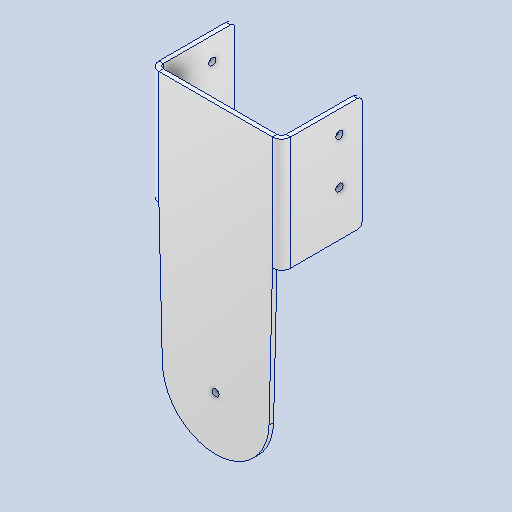
# Autodesk Inventor part: servoplate2_forR3
Saved by Autodesk Inventor 2024.3 (Build 283343010, 343A)
## iProperties
Created: 2025-05-28
Part Number: servoplate2_forR3
Material: アルミニウム 6061
Document SubType Name: Sheet Metal
Designer: kshau
Density: 2.7 g/cm^3
Sheet Metal Rule: Default
Appearance: アルミニウム - フラット
Mass: 54.6317 g
Surface Area: 213.118 cm^2
Volume: 20.234 cm^3
Flat Pattern Width: 13.35 cm
Flat Pattern Length: 12.2048 cm
Flat Pattern Area: 162.934 cm^2
Sheet Metal Width: 133.500 mm
Sheet Metal Length: 122.048 mm
Sheet Metal Area: 16293.380 mm^2
Author: kshau
Autodesk Inventor part; units mm, degrees
ref_plane "YZ Plane" through (0, 0, 0) normal (1, 0, 0) x (0, 1, 0)
ref_plane "XZ Plane" through (0, 0, 0) normal (0, 1, 0) x (-1, 0, 0)
ref_plane "XY Plane" through (0, 0, 0) normal (0, 0, 1) x (1, 0, 0)
sketch "スケッチ1" plane through (0, 0, 0) normal (0, 0, 1) x (1, 0, 0)
  circle A0 centre (0, 0) radius 23.5
  line L0 (0, 0) -> (0, 60)
  line L1 (0, 60) -> (25, 60)
  line L2 (25, 60) -> (25, 110)
  line L3 (25, 110) -> (0, 110)
  line L4 (0, 110) -> (0, 60)
  line L5 (25, 60) -> (23.4927, -0.5845)
  line L6 (0, 60) -> (-25, 60)
  line L7 (-25, 60) -> (-25, 110)
  line L8 (-25, 110) -> (0, 110)
  line L9 (-25, 60) -> (-23.4927, -0.5845)
  point P0 (-23.4927, -0.5845)
  dimension "d0" = 47
  dimension "d1" = 60
  dimension "d2" = 50
  dimension "d3" = 25
  measures "d1" distance of L0.start L0.end
  measures "d2" distance of L1.end L2.end
  measures "d3" distance of L0.end L1.end
extrude "プレート1" add sketch "スケッチ1" along normal blind 2
sketch "スケッチ2" plane through (27, 60, -2) normal (1, 0, 0) x (0, 1, 0)
  line L0 (50, 0) -> (0, 0)
  line L1 (0, 0) -> (0, -31.5)
  line L2 (0, -31.5) -> (50, -31.5)
  line L3 (50, -31.5) -> (50, 0)
  constraints: 6 end point, 1 horizontal, 1 perpendicular, 1 vertical
edge flange "フランジ1" height 35.5 angle 90 thickness 2 bend radius 2 thickness toward (1, 0, 0) relief straight relief width 2 relief depth 1 edges at (25, 85, 0) wall of the first edge with corners at (27, 110, -2) (27, 60, -2) (27, 60, -33.5) (27, 110, -33.5)
bend "曲げ1"
corner "コーナー1"
sketch "スケッチ3" plane through (-27, 110, -2) normal (-1, 0, 0) x (0, -1, 0)
  line L0 (50, 0) -> (0, 0)
  line L1 (0, 0) -> (0, -31.5)
  line L2 (0, -31.5) -> (50, -31.5)
  line L3 (50, -31.5) -> (50, 0)
  constraints: 6 end point, 1 horizontal, 1 perpendicular, 1 vertical
edge flange "フランジ2" height 35.5 angle 90 thickness 2 bend radius 2 thickness toward (-1, 0, 0) relief straight relief width 2 relief depth 1 edges at (-25, 85, 0) wall of the first edge with corners at (-27, 60, -2) (-27, 110, -2) (-27, 110, -33.5) (-27, 60, -33.5)
bend "曲げ2"
corner "コーナー2"
sketch "スケッチ4" plane through (0, 0, 2) normal (0, 0, 1) x (1, 0, 0)
  circle A0 centre (0, 0) radius 10.1
  dimension "d25" = 20.2
  constraints: 1 centre point, 1 coincident
  measures "d25" diameter of A0
extrude "押し出し1" [suppressed]
sketch "スケッチ5" plane through (0, 0, 2) normal (0, 0, 1) x (1, 0, 0)
  circle A0 centre (0, 0) radius 15.18
  point P0 (0, 15.18)
  point P1 (-13.1463, 7.59)
  point P2 (-13.1463, -7.59)
  point P3 (0, -15.18)
  point P4 (13.1463, -7.59)
  point P5 (13.1463, 7.59)
  dimension "d28" = 30.36
  dimension "d31" = 360
  constraints: 1 coincident, 1 vertical alignment, 9 other
hole "穴1" [suppressed]
sketch "スケッチ6" plane through (29, 60, -33.5) normal (1, 0, 0) x (0, 0, -1)
  line L0 (0, 0) -> (0, 50) projected
  line L1 (0, 10) -> (-31.5, 10)
  line L2 (-31.5, 50) -> (-31.5, 0) projected
  line L3 (0, 0) -> (-31.5, 0) projected
  line L4 (0, 50) -> (-31.5, 50) projected
  line L5 (-10, 50) -> (-10, 10)
  point P0 (-33.5, -60)
  point P1 (-10, 20)
  point P2 (-10, 40)
  point P3 (-33.5, 50)
  dimension "d40" = 10
  dimension "d42" = 10
  dimension "d43" = 20
  dimension "d69" = 23.5
  constraints: 6 point on line, 4 end point, 1 horizontal, 1 perpendicular
  measures "d40" distance between parallel lines of L3 L1
  measures "d42" distance from line of L1 point (-10, 20)
  measures "d43" distance of point (-10, 20) point (-10, 40)
  measures "d69" distance from line of L5 point (-33.5, 50)
hole "穴2" at (29, 80, -23.5) at (29, 100, -23.5) direction (-1, 0, 0) diameter 3.2 end through all
sketch "スケッチ7" plane through (0, 0, 0) normal (0, 0, -1) x (-1, 0, 0)
  point P0 (0, 0)
  point P1 (0, 0)
  constraints: 1 coincident
hole "穴3" at (0, 0, 0) direction (0, 0, 1) diameter 3.1 end through all
sketch "スケッチ8" plane through (0, 0, 2) normal (0, 0, 1) x (1, 0, 0)
  line L0 (-15, 100) -> (15, 100)
  line L1 (15, 100) -> (15, 60)
  line L2 (15, 60) -> (-15, 60)
  line L3 (-15, 60) -> (-15, 100)
  line L4 (25, 110) -> (25, 60) projected
  line L5 (-25, 60) -> (-25, 110) projected
  line L6 (-25, 110) -> (25, 110) projected
  circle A0 centre (0, 0) radius 1.55 projected
  circle A1 centre (0, 0) radius 13.5
  line L7 (-14.4993, 40) -> (-13.4958, -0.3358)
  line L8 (-23.4927, -0.5845) -> (-25, 60) projected
  line L9 (13.4958, -0.3358) -> (14.4993, 40)
  line L10 (25, 60) -> (23.4927, -0.5845) projected
  line L11 (14.4993, 40) -> (-14.4993, 40)
  dimension "d58" = 10
  dimension "d59" = 10
  dimension "d60" = 10
  dimension "d61" = 40
  dimension "d63" = 10
  dimension "d64" = 20
  constraints: 14 end point, 5 parallel, 2 point on circle, 2 tangent, 1 centre point, 1 coincident, 1 horizontal, 1 perpendicular
  measures "d58" distance between parallel lines of L4 L1
  measures "d59" distance between parallel lines of L5 L3
  measures "d60" distance between parallel lines of L6 L0
  measures "d61" distance between parallel lines of L0 L2
  measures "d63" distance between parallel lines of L8 L7
  measures "d64" distance between parallel lines of L2 L11
extrude "押し出し2" [suppressed]
fillet "フィレット1" [suppressed]
fillet "フィレット2" radius 2 4 edges at (28, 110, -33.5) (28, 60, -33.5) (-28, 60, -33.5) (-28, 110, -33.5)
equation "\"d38\" = Thickness"
equation "\"d56\" = Thickness"
equation "\"d4\" = Thickness"
equation "\"d5\" = BendReliefWidth"
equation "\"d6\" = BendReliefDepth"
equation "\"d7\" = MinimumRemnant"
equation "\"d8\" = TransitionRadius"
equation "\"d11\" = BendRadius"
equation "\"d12\" = CornerReliefSize"
equation "\"d13\" = GapSize"
equation "\"d14\" = JacobiRadiusSize"
equation "\"d15\" = BendReliefWidth"
equation "\"d16\" = BendReliefDepth"
equation "\"d17\" = MinimumRemnant"
equation "\"d18\" = TransitionRadius"
equation "\"d21\" = BendRadius"
equation "\"d22\" = CornerReliefSize"
equation "\"d23\" = GapSize"
equation "\"d24\" = JacobiRadiusSize"
equation "\"BendRadius\" = Thickness"
equation "\"BendReliefWidth\" = Thickness"
equation "\"BendReliefDepth\" = 0.5 * Thickness"
equation "\"CornerReliefSize\" = 4 * Thickness"
equation "\"MinimumRemnant\" = 2 * Thickness"
equation "\"TransitionRadius\" = BendRadius"
equation "\"JacobiRadiusSize\" = BendRadius"
equation "\"GapSize\" = Thickness"
equation "\"Thickness\" = 2"
